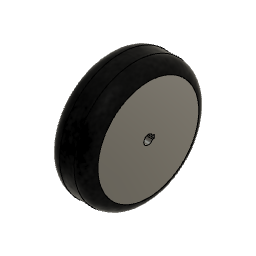
wheel (Autodesk Fusion 360 design; units mm, degrees)
Autodesk Fusion 360 part; units mm, degrees
sketch "Sketch1" plane through (0, 0, 0) normal (1, 0, 0) x (0, 1, 0)
  circle A0 centre (0, 0) radius 94.3
  circle A1 centre (0, 0) radius 8.5
  line L0 (2.9756, 10.9) -> (-3.0244, 10.9)
  line L1 (-3.0244, 10.9) -> (-3.0244, 6.1)
  line L2 (-3.0244, 6.1) -> (2.9756, 6.1)
  line L3 (2.9756, 6.1) -> (2.9756, 10.9)
  line L4 (2.9756, 10.9) -> (-3.0244, 6.1) construction
  line L5 (-3.0244, 10.9) -> (2.9756, 6.1) construction
  point P0 (-0.0244, 8.5)
  dimension "d1" = 188.6
  dimension "d2" = 17
  dimension "d3" = 6
  dimension "d4" = 4.8
  constraint coincident A0.centre A1.centre
  constraint concentric A0 A1
  constraint horizontal L0
  constraint perpendicular L0 L1
  constraint parallel L0 L2
  constraint parallel L1 L3
  constraint coincident L4 P0
  constraint coincident L5 P0
  constraint coincident A1 P0
  measures "d1" diameter of A0
  measures "d2" diameter of A1
  measures "d3" distance of L1.end L2.end
  measures "d4" distance of L0.end L1.end
extrude "Extrude1" add sketch "Sketch1" along normal blind 76 makes body 1
move_body "Move1" bodies 1 to x (1, 0, 0) y (0, 1, 0) z (0, 0, 1) at (-38, 0, 0)
sketch "Sketch2" plane through (38, 0, 0) normal (1, 0, 0) x (0, 1, 0)
  arc A0 (-3.0244, 7.9437) -> (2.9756, 7.9622) centre (0, 0) ccw
  line L0 (-3.0244, 7.9437) -> (-3.0244, 10.9)
  line L1 (-3.0244, 10.9) -> (2.9756, 10.9)
  line L2 (2.9756, 10.9) -> (2.9756, 7.9622)
  circle A1 centre (0, 0) radius 94.3
  circle A2 centre (0, 0) radius 114.3
  circle A3 centre (0, 0) radius 94.3
  dimension "d7" = 228.6
  constraint concentric A0 A2
  constraint concentric A0 A3
  measures "d7" diameter of A2
extrude "Extrude2" add sketch "Sketch2" against normal blind 76 separate body contours A2 makes body 2
fillet "Fillet1" radius 25 1 edges at (38, -106.565, -41.3326) on bodies 2
fillet "Fillet2" radius 25 1 edges at (-38, -106.565, 41.3326) on bodies 2
copy_body "Body->Comp1" bodies 1 removing the originals makes body 3 in component "wheel"
copy_body "CutPasteBodies1" bodies 2 removing the originals makes body 4 in component "wheel"
component "wheel" placed x (1, 0, 0) y (0, 1, 0) z (0, 0, 1) at (0, 0, 0)
named bodies: "rim", "tire"
